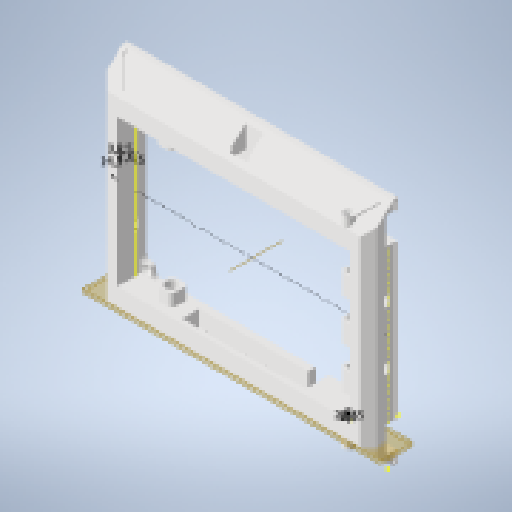
# Autodesk Inventor part: up_part
Saved by Autodesk Inventor 2025 (Build 290162000, 162)
## iProperties
Created: 2026-07-31
Part Number: up_part
Material: Типовые
Document SubType Name: Modeling
Designer: garin
Density: 1 g/cm^3
Appearance: По умолчанию
Author: garin
Autodesk Inventor part; units mm, degrees
ref_plane "YZ Plane" through (0, 0, 0) normal (1, 0, 0) x (0, 1, 0)
ref_plane "XZ Plane" through (0, 0, 0) normal (0, 1, 0) x (-1, 0, 0)
ref_plane "XY Plane" through (0, 0, 0) normal (0, 0, 1) x (1, 0, 0)
sketch "Эскиз1" plane through (0, 0, 0) normal (0, 0, 1) x (1, 0, 0)
  line L0 (0, 0) -> (-157, 0)
  line L1 (-157, 0) -> (-157, 133.4)
  line L2 (-157, 133.4) -> (0, 133.4)
  line L3 (0, 133.4) -> (0, 0)
  line L4 (-157, 66.7) -> (0, 66.7) construction
  line L5 (-78.5, 0) -> (-78.5, 133.4) construction
  line L6 (-11, 24.1) -> (-146, 24.1)
  line L7 (-146, 24.1) -> (-146, 109.3)
  line L8 (-146, 109.3) -> (-11, 109.3)
  line L9 (-11, 109.3) -> (-11, 24.1)
  line L10 (-11, 24.1) -> (-146, 109.3) construction
  line L11 (-146, 24.1) -> (-11, 109.3) construction
  line L12 (0, 0) -> (-2, 0) construction
  line L13 (-2, 0) -> (-2, 54.105) construction
  line L14 (-2, 54.105) -> (0, 54.105) construction
  line L15 (0, 54.105) -> (0, 0) construction
  line L16 (-2, 54.105) -> (-2, 73.295)
  line L17 (-2, 73.295) -> (-11, 73.295)
  line L18 (-2, 54.105) -> (-11, 54.105)
  line L19 (-157, 133.4) -> (-137, 133.4) construction
  line L20 (-157, 110.4) -> (-157, 133.4) construction
  line L21 (-157, 0) -> (-140, 0)
  line L22 (-140, 0) -> (-140, 22)
  line L23 (-140, 22) -> (-157, 22)
  line L24 (-157, 22) -> (-157, 0)
  line L25 (-157, 0) -> (-140, 0)
  line L26 (-140, 0) -> (-140, 6.5)
  line L27 (-140, 6.5) -> (-157, 6.5)
  line L28 (-157, 6.5) -> (-157, 0)
  line L29 (-140, 133.4) -> (-140, 111.4)
  line L30 (-140, 111.4) -> (-157, 111.4)
  line L31 (-140, 126.9) -> (-157, 126.9)
  line L32 (-17, 0) -> (-17, 22)
  line L33 (-17, 22) -> (0, 22)
  line L34 (-17, 6.5) -> (0, 6.5)
  line L35 (-17, 111.4) -> (0, 111.4)
  line L36 (-17, 126.9) -> (0, 126.9)
  line L37 (-17, 133.4) -> (-17, 111.4)
  point P0 (-78.5, 66.7)
  point P1 (0, 111.4)
  point P2 (0, 126.9)
  point P3 (-17, 126.9)
  point P4 (-140, 126.9)
  point P5 (0, 6.5)
  dimension "d0" = 157
  dimension "d1" = 133.4
  dimension "d2" = 135
  dimension "d3" = 85.2
  dimension "d20" = 2
  dimension "d21" = 54.105
  dimension "d22" = 19.19
  dimension "d75" = 17
  dimension "d76" = 22
  dimension "d77" = 17
  dimension "d78" = 6.5
  constraints: 76 end point, 15 symmetric about line, 10 parallel, 7 midpoint, 7 perpendicular, 6 horizontal, 2 point on line, 1 vertical
  measures "d0" distance of L1.end L2.end
  measures "d1" distance of L0.end L1.end
  measures "d2" distance of L7.end L8.end
  measures "d3" distance of L6.end L7.end
  measures "d20" distance of L13.end L14.end
  measures "d21" distance of L12.end L13.end
  measures "d22" distance of L13.end L16.end
  measures "d75" distance of L23.end L22.end
  measures "d76" distance of L22.end L21.end
  measures "d77" distance of L27.end L26.end
  measures "d78" distance of L26.end L25.end
extrude "Выдавливание1" add sketch "Эскиз1" along normal blind 17 contours L0 L32 L34 L3 | L0 L22 L23 L1 L30 L29 L2 L37 L35 L3 L33 L32 | L34 L32 L33 L3 | L0 L1 L27 L22 | L27 L1 L23 L22 | L35 L37 L36 L3 | L36 L37 L2 L3 | L1 L31 L29 L30 | L1 L2 L29 L31 | L9 L17 L16 L18
chamfer "Фаска1" distance 14 angle 45 2 edges at (-78.5, 0, 17) (-78.5, 133.4, 17)
chamfer "Фаска2" distance 5 angle 45 2 edges at (-157, 66.7, 17) (0, 66.7, 17)
sketch "Эскиз2" plane through (-157, 0, 3) normal (0, -0.7071068, 0.7071068) x (1, 0, 0)
  line L0 (0, -2.1213) -> (157, -2.1213) projected
  line L1 (0, -2.1213) -> (157, -2.1213)
  line L2 (157, -2.1213) -> (157, 19.7987)
  line L3 (157, 19.7987) -> (0, 19.7987)
  line L4 (0, 19.7987) -> (0, -2.1213)
  line L5 (78.5, 19.7987) -> (78.5, -2.1213) construction
  line L6 (0, 8.8387) -> (157, 8.8387) construction
  line L7 (154, 1.3387) -> (3, 1.3387) construction
  line L8 (3, 1.3387) -> (3, 16.3387) construction
  line L9 (3, 16.3387) -> (154, 16.3387) construction
  line L10 (154, 16.3387) -> (154, 1.3387) construction
  line L11 (154, 1.3387) -> (3, 16.3387) construction
  line L12 (3, 1.3387) -> (154, 16.3387) construction
  line L13 (3, 16.3387) -> (12, 16.3387) construction
  line L14 (12, 16.3387) -> (3, 3.6108)
  line L15 (0, 12.7279) -> (5, 19.799) construction
  line L16 (145, 16.3387) -> (154, 3.6108)
  line L17 (12, 16.3387) -> (145, 16.3387)
  line L18 (11, 14.92) -> (11, 26.9408) projected
  line L19 (154, 3.6108) -> (154, 1.3387)
  line L20 (154, 1.3387) -> (3, 1.3387)
  line L21 (3, 3.6108) -> (3, 1.3387)
  line L22 (5.2571, 3.3387) -> (13.0353, 14.3387)
  line L23 (13.0353, 14.3387) -> (143.9647, 14.3387)
  line L24 (143.9647, 14.3387) -> (151.7429, 3.3387)
  line L25 (151.7429, 3.3387) -> (5.2571, 3.3387)
  point P0 (78.5, 8.8387)
  dimension "d12" = 157
  dimension "d13" = 21.92
  dimension "d14" = 151
  dimension "d15" = 15
  dimension "d16" = 9
  dimension "d17" = 2
  constraints: 46 end point, 7 midpoint, 5 parallel, 5 perpendicular, 2 horizontal, 2 point on line, 2 symmetric about line, 1 collinear, 3 other
  measures "d12" distance of L3.end L2.end
  measures "d13" distance of L2.end L1.end
  measures "d14" distance of L8.end L9.end
  measures "d15" distance of L7.end L8.end
  measures "d16" distance of L8.end L13.end
  measures "d17" distance between parallel lines of L14 L22
extrude "Выдавливание2" cut sketch "Эскиз2" against normal blind 1 contours L17 L16 L19 L20 L21 L14
ref_plane "РабПлоскость1" through (-157, 66.7, 0) normal (0, 1, 0) x (1, 0, 0)
mirror "Зеркальное отражение1" about plane through (-157, 66.7, 0) normal (0, 1, 0) of "Выдавливание2"
extrude "Выдавливание3" cut sketch "Эскиз1" along normal blind 11.1 contours L9 L17 L16 L18
sketch "Эскиз3" plane through (-157, 0, 0) normal (0, -1, 0) x (1, 0, 0)
  line L0 (0, 0) -> (157, 0) construction
  line L1 (0, 0) -> (157, 0) construction
  line L2 (157, 0) -> (157, 17) construction
  line L3 (157, 17) -> (0, 17) construction
  line L4 (0, 17) -> (0, 0) construction
  line L5 (78.5, 17) -> (78.5, 0) construction
  line L6 (0, 8.5) -> (157, 8.5) construction
  line L7 (145, 14.5532) -> (12, 14.5532) construction
  line L8 (12, 14.5532) -> (12, 3.9466) construction
  line L9 (3, 3.9466) -> (154, 3.9466) construction
  line L10 (12, 9.2499) -> (78.5, 9.2499) construction
  line L11 (12, 9.2499) -> (78.5, 9.2499) construction
  line L12 (83.5, 4.2499) -> (73.5, 4.2499)
  line L13 (73.5, 4.2499) -> (73.5, 14.2499)
  line L14 (73.5, 14.2499) -> (83.5, 14.2499)
  line L15 (83.5, 14.2499) -> (83.5, 4.2499)
  line L16 (83.5, 4.2499) -> (73.5, 14.2499) construction
  line L17 (73.5, 4.2499) -> (83.5, 14.2499) construction
  line L18 (46.5, 13.7499) -> (108.5, 13.7499) construction
  line L19 (108.5, 13.7499) -> (108.5, 4.7499) construction
  line L20 (108.5, 4.7499) -> (46.5, 4.7499) construction
  line L21 (46.5, 4.7499) -> (46.5, 13.7499) construction
  line L22 (46.5, 13.7499) -> (108.5, 4.7499) construction
  line L23 (108.5, 13.7499) -> (46.5, 4.7499) construction
  line L24 (109, 14.2499) -> (46, 14.2499)
  line L25 (46, 14.2499) -> (46, 4.2499)
  line L26 (46, 4.2499) -> (109, 4.2499)
  line L27 (109, 4.2499) -> (109, 14.2499)
  line L28 (46.5, 9.2499) -> (48.3, 9.2499) construction
  line L29 (48.3, 7.2499) -> (48.3, 11.2499) construction
  circle A0 centre (48.3, 11.2499) radius 1.75
  circle A1 centre (48.3, 7.2499) radius 1.75
  line L30 (109, 14.2499) -> (117, 14.2499)
  line L31 (117, 14.2499) -> (117, 4.2499)
  line L32 (117, 4.2499) -> (109, 4.2499)
  line L33 (109, 4.2499) -> (109, 14.2499)
  line L34 (108.5, 13.7499) -> (98.75, 13.7499) construction
  line L35 (98.75, 13.7499) -> (98.75, 11.6499) construction
  line L36 (98.75, 11.6499) -> (108.5, 11.6499) construction
  line L37 (108.5, 11.6499) -> (108.5, 13.7499) construction
  circle A2 centre (98.75, 11.6499) radius 1.75
  line L38 (78.5, 9.2499) -> (77.5, 9.2499) construction
  line L39 (97, 11.6499) -> (97, 14.2499) construction
  line L40 (97, 14.2499) -> (95.5, 14.2499) construction
  line L41 (95.5, 14.2499) -> (95.5, 4.2499)
  line L42 (95.5, 4.2499) -> (97, 4.2499) construction
  line L43 (97, 4.2499) -> (97, 14.2499) construction
  line L44 (83.5, 14.2499) -> (84.5, 14.2499) construction
  line L45 (84.5, 14.2499) -> (84.5, 4.2499)
  line L46 (84.5, 4.2499) -> (83.5, 4.2499) construction
  line L47 (83.5, 4.2499) -> (83.5, 14.2499) construction
  line L48 (73.5, 14.2499) -> (71.5, 14.2499) construction
  line L49 (71.5, 14.2499) -> (71.5, 4.2499)
  line L50 (71.5, 4.2499) -> (73.5, 4.2499) construction
  line L51 (73.5, 4.2499) -> (73.5, 14.2499) construction
  line L52 (46, 14.2499) -> (50.15, 14.2499) construction
  line L53 (50.15, 14.2499) -> (50.15, 4.2499)
  line L54 (50.15, 4.2499) -> (46, 4.2499) construction
  line L55 (46, 4.2499) -> (46, 14.2499) construction
  line L56 (117, 4.2499) -> (109, 4.2499)
  line L57 (109, 4.2499) -> (109, -0.0001)
  line L58 (109, -0.0001) -> (117, -0.0001)
  line L59 (117, -0.0001) -> (117, 4.2499)
  point P0 (50.15, 14.2499)
  point P1 (50.15, 4.2499)
  point P2 (71.5, 4.2499)
  point P3 (71.5, 14.2499)
  dimension "d41" = 3.5
  dimension "d25" = 157
  dimension "d26" = 17
  dimension "d28" = 10
  dimension "d29" = 10
  dimension "d30" = 62
  dimension "d31" = 9
  dimension "d32" = 0.5
  dimension "d33" = 1.8
  dimension "d34" = 4
  dimension "d35" = 3.5
  dimension "d36" = 3.5
  dimension "d37" = 8
  dimension "d38" = 10
  dimension "d39" = 9.75
  dimension "d40" = 2.1
  dimension "d42" = 1
  dimension "d44" = 1.5
  dimension "d45" = 10
  dimension "d46" = 1
  dimension "d47" = 10
  dimension "d48" = 2
  dimension "d49" = 10
  dimension "d50" = 4.15
  dimension "d51" = 10
  dimension "d63" = 8
  dimension "d64" = 4.25
  constraints: 114 end point, 23 parallel, 12 horizontal, 12 perpendicular, 11 midpoint, 8 point on line, 3 coincident, 3 vertical, 2 centre point, 1 collinear, 1 horizontal alignment, 5 other
  measures "d25" distance of L3.end L2.end
  measures "d26" distance of L2.end L1.end
  measures "d28" distance of L13.end L14.end
  measures "d29" distance of L12.end L13.end
  measures "d30" distance of L19.end L20.end
  measures "d31" distance of L18.end L19.end
  measures "d32" distance between parallel lines of L18 L24
  measures "d33" distance of L28.end L28.start
  measures "d34" distance of L29.start L29.end
  measures "d35" diameter of A0
  measures "d36" diameter of A1
  measures "d37" distance of L31.end L32.end
  measures "d38" distance of L30.end L31.end
  measures "d39" distance of L36.end L35.end
  measures "d40" distance of L35.end L34.end
  measures "d42" distance of L11.end L38.end
  measures "d44" distance of L42.end L41.end
  measures "d45" distance of L41.end L40.end
  measures "d46" distance of L45.end L46.end
  measures "d47" distance of L44.end L45.end
  measures "d48" distance of L50.end L49.end
  measures "d49" distance of L49.end L48.end
  measures "d50" distance of L53.end L54.end
  measures "d51" distance of L52.end L53.end
  measures "d63" distance of L58.end L57.end
  measures "d64" distance of L57.end L56.end
extrude "Выдавливание4" cut sketch "Эскиз3" along normal blind 25 from surface at -24.1 contours L12 L13 L14 L15
ref_plane "РабПлоскость4" through (-145, 12.2603, 13.8461) normal (0, 1, 0) x (1, 0, 0)
ref_plane "РабПлоскость5" through (-145, 15.0603, 13.8461) normal (0, 1, 0) x (1, 0, 0)
extrude "Выдавливание5" cut sketch "Эскиз3" against normal blind 13 from surface at -12.2603 contours L27 L30 L31 L32 | L32 L59 L58 L57
extrude "Выдавливание6" cut sketch "Эскиз3" against normal blind 10 from surface at -15.0603 contours L12 L13 L14 L15 | L15 L24 L45 L26 | L26 L49 L24 L13 | L45 L24 L41 L26 | L26 L53 L24 L49 | L41 L24 L27 L26 | L26 L25 L24 L53 | A0 | A1 | A2
extrude "Выдавливание7" cut sketch "Эскиз3" along normal blind 3 from surface at -15.0603 contours A0 | A1 | A2
extrude "Выдавливание8" cut sketch "Эскиз3" along normal blind 2 from surface at -15.0603 contours L45 L24 L41 L26 | L26 L53 L24 L49
pattern_circular "Круговой массив1" count 2 over 360 about axis through (-78.5, 66.7, 0) along (0, 0, -1) of "Выдавливание4", "Выдавливание8", "Выдавливание6", "Выдавливание7", "Выдавливание5"
chamfer "Фаска3" distance 2 angle 45 1 edges at (-2, 63.7, 11.1)
sketch "Эскиз5" plane through (0, 0, 0) normal (1, 0, 0) x (0, 0, -1)
  line L0 (-12, 9) -> (-12, 124.4) projected
  line L1 (-3, 0) -> (-12, 9) projected
  line L2 (0, 0) -> (-3, 0) projected
  line L3 (0, 0) -> (0, 133.4) projected
  line L4 (0, 133.4) -> (-3, 133.4) projected
  line L5 (-12, 124.4) -> (-3, 133.4) projected
  line L6 (-11, 123.9858) -> (-11, 9.4142)
  line L7 (-11, 9.4142) -> (-2.5858, 1)
  line L8 (-2.5858, 1) -> (-1, 1)
  line L9 (-1, 1) -> (-1, 132.4)
  line L10 (-1, 132.4) -> (-2.5858, 132.4)
  line L11 (-2.5858, 132.4) -> (-11, 123.9858)
  line L12 (-10, 9.8284) -> (-10, 123.5716)
  line L13 (-10, 123.5716) -> (-2, 131.5716)
  line L14 (-2, 131.5716) -> (-2, 1.8284)
  line L15 (-2, 1.8284) -> (-10, 9.8284)
  dimension "d81" = 1
  dimension "d82" = 1
  constraints: 20 end point, 8 other
  measures "d81" distance between parallel lines of L0 L6
  measures "d82" distance between parallel lines of L6 L12
extrude "Выдавливание11" cut sketch "Эскиз1" along normal blind 6 contours L34 L32 L33 L3 | L27 L1 L23 L22 | L35 L37 L36 L3 | L1 L31 L29 L30
extrude "Выдавливание12" cut sketch "Эскиз5" against normal blind 1 contours L11 L10 L9 L8 L7 L6 | L12 L13 L14 L15
chamfer "Фаска4" distance 1 angle 45 4 edges at (-9, 6.5, 6) (-9, 126.9, 6) (-148.5, 126.9, 6) (-148.5, 6.5, 6)
ref_plane "РабПлоскость6" through (-78.5, 22, 0) normal (1, 0, 0) x (0, 0, -1)
mirror "Зеркальное отражение3" about plane through (-78.5, 22, 0) normal (1, 0, 0) of "Выдавливание12"
ref_plane "РабПлоскость7" through (0, 0, 6) normal (0, 0, 1) x (1, 0, 0)
sketch "Эскиз6" plane through (0, 0, 6) normal (0, 0, 1) x (1, 0, 0)
  line L0 (0, 111.4) -> (0, 22) construction
  line L1 (0, 66.7) -> (-157, 66.7) construction
  line L2 (-157, 124.4) -> (-157, 9) construction
  line L3 (-157, 66.7) -> (-157, 81.2) construction
  line L4 (-146, 24.1) -> (-146, 109.3) construction
  line L5 (-157, 81.2) -> (-146, 81.2) construction
  line L6 (-146, 81.2) -> (-146, 86.2) construction
  line L7 (-146, 86.2) -> (-157, 86.2) construction
  line L8 (-157, 86.2) -> (-157, 81.2) construction
  line L9 (-157, 83.7) -> (-146, 83.7) construction
  line L10 (-157, 83.7) -> (-148.5, 83.7) construction
  circle A0 centre (-148.5, 83.7) radius 0.8
  circle A1 centre (-148.5, 49.7) radius 0.8
  line L11 (-157, 81.2) -> (-157, 81) construction
  line L12 (-157, 81) -> (-146, 81)
  line L13 (-157, 86.4) -> (-146, 86.4)
  line L14 (-146, 86.4) -> (-146, 81)
  line L15 (-146, 24.1) -> (-146, 109.3) projected
  line L16 (-157, 81) -> (-157, 86.4)
  line L17 (-157, 52.4) -> (-146, 52.4)
  line L18 (-157, 47) -> (-146, 47)
  line L19 (-146, 47) -> (-146, 52.4)
  line L20 (-157, 52.4) -> (-157, 47)
  point P0 (0, 0)
  dimension "d91" = 14.5
  dimension "d92" = 5
  dimension "d93" = 8.5
  dimension "d94" = 1.6
  dimension "d99" = 0.2
  constraints: 34 end point, 7 symmetric about line, 5 point on line, 4 midpoint, 2 centre point, 2 collinear, 2 parallel, 2 perpendicular, 1 coincident, 1 horizontal, 1 other
  measures "d91" distance of L1.end L3.end
  measures "d92" distance of L6.end L5.end
  measures "d93" distance of L9.start L10.end
  measures "d94" diameter of A0
  measures "d99" distance of L3.end L11.end
extrude "Выдавливание13" cut sketch "Эскиз6" along normal blind 4 and the other way blind 6 contours A0 | A1
extrude "Выдавливание14" cut sketch "Эскиз6" along normal mid plane 2.8 contours A0 | A1 | L16 L13 L14 L12 | L18 L20 L17 L15
chamfer "Фаска5" distance 0.9 angle 45 2 edges at (-149.3, 83.7, 0) (-149.3, 49.7, 0)
mirror "Зеркальное отражение4" about plane through (-78.5, 22, 0) normal (1, 0, 0) of "Выдавливание14", "Выдавливание13", "Фаска5"
ref_plane "РабПлоскость8" through (-146, 36.9, 17) normal (0, 1, 0) x (1, 0, 0)
sketch "Эскиз7" plane through (-146, 24.1, 17) normal (0, 1, 0) x (1, 0, 0)
  line L0 (135, 17) -> (135, 0) projected
  line L1 (135, 0) -> (131.45, 0) construction
  line L2 (131.45, 0) -> (131.45, 2.95) construction
  line L3 (131.45, 2.95) -> (135, 2.95) construction
  line L4 (135, 2.95) -> (135, 0) construction
  circle A0 centre (131.45, 2.95) radius 1.3
  circle A1 centre (131.45, 2.95) radius 2.95
  line L5 (131.45, 5.9) -> (135, 5.9)
  line L6 (135, 5.9) -> (135, 0)
  line L7 (131.45, 0) -> (135, 0)
  circle A2 centre (131.45, 2.95) radius 3.5
  point P0 (146, 17)
  dimension "d105" = 3.55
  dimension "d106" = 2.95
  dimension "d107" = 2.6
  dimension "d117" = 7
  constraints: 14 end point, 3 centre point, 3 coincident, 3 equal length, 3 perpendicular, 2 point on circle, 2 tangent, 1 horizontal, 1 point on line
  measures "d105" distance of L2.end L3.end
  measures "d106" distance of L1.end L2.end
  measures "d107" diameter of A0
  measures "d117" diameter of A2
extrude "Выдавливание15" add sketch "Эскиз7" along normal blind 11.6 from surface at 12.8 contours L0 L7 A2 L5 | A2 L7 A1 L5 | A1 picked at (134.7433, 3.1824)
pattern_linear "Прямоуг.массив1" count 3 spacing 24 along (0, 1, 0) of "Выдавливание15"
fillet "Сопряжение2" radius 2 2 edges at (-11, 42.7, 11.1) (-11, 90.7, 11.1)
ref_plane "РабПлоскость10" through (-5, 14, 17) normal (0, 1, 0) x (1, 0, 0)
extrude "Выдавливание16" cut sketch "Эскиз7" against normal blind 20 contours A0
extrude "Выдавливание17" add sketch "Эскиз7" against normal blind 5.9 from surface at -10.1 contours A1
chamfer "Фаска6" distance 1.65 angle 45 1 edges at (-15.85, 8.1, 14.05)
mirror "Зеркальное отражение5" about plane through (-157, 66.7, 0) normal (0, 1, 0) of "Выдавливание17", "Фаска6", "Выдавливание16"
sketch "Эскиз9" plane through (-146, 24.1, 17) normal (0, 1, 0) x (1, 0, 0)
  line L0 (106, 3.1539) -> (106, 2.7501) projected
  line L1 (106, 17) -> (106, 3.1539) projected
  line L2 (106, 2.7501) -> (106, 17)
  line L3 (39.15, 2.7501) -> (35, 2.7501) projected
  line L4 (35, 2.7501) -> (35, 17) construction
  line L5 (-11, 17) -> (146, 17) projected
  line L6 (35, 9.8751) -> (22, 9.8751) construction
  line L7 (27, 4.8751) -> (17, 4.8751)
  line L8 (17, 4.8751) -> (17, 14.8751)
  line L9 (17, 14.8751) -> (27, 14.8751)
  line L10 (27, 14.8751) -> (27, 4.8751)
  line L11 (27, 4.8751) -> (17, 14.8751) construction
  line L12 (17, 4.8751) -> (27, 14.8751) construction
  circle A0 centre (22, 9.8751) radius 3.6
  dimension "d135" = 13
  dimension "d136" = 10
  dimension "d137" = 10
  dimension "d138" = 7.2
  constraints: 18 end point, 3 midpoint, 2 horizontal, 2 parallel, 1 centre point, 1 coincident, 1 collinear, 1 perpendicular, 1 point on line, 1 vertical
  measures "d135" distance of L6.start L6.end
  measures "d136" distance of L8.end L9.end
  measures "d137" distance of L7.end L8.end
  measures "d138" diameter of A0
extrude "Выдавливание19" add sketch "Эскиз9" along normal blind 7
fillet "Сопряжение3" radius 3 4 edges at (-129, 27.6, 12.1249) (-129, 27.6, 2.1249) (-119, 27.6, 12.1249) (-119, 27.6, 2.1249)
mirror "Зеркальное отражение6" about plane through (-157, 66.7, 0) normal (0, 1, 0) of "Сопряжение3", "Выдавливание19"
sketch "Эскиз10" plane through (0, 0, 0) normal (0, 0, -1) x (-1, 0, 0)
  line L0 (146, 109.3) -> (11, 109.3) projected
  line L1 (146, 109.3) -> (140, 109.3)
  line L2 (140, 109.3) -> (140, 103.3)
  line L3 (140, 103.3) -> (146, 103.3)
  line L4 (146, 103.3) -> (146, 109.3)
  line L5 (143, 109.3) -> (143, 103.3) construction
  line L6 (140, 106.3) -> (146, 106.3) construction
  circle A0 centre (143, 106.3) radius 1.25
  line L7 (78.5, 109.3) -> (78.5, 24.1) construction
  line L8 (48, 24.1) -> (146, 24.1) construction
  line L9 (13.25, 72.5) -> (13.25, 60.9) construction
  line L10 (13.25, 66.7) -> (146, 66.7) construction
  line L11 (146, 24.1) -> (146, 109.3) construction
  line L12 (11, 109.3) -> (17, 109.3)
  line L13 (17, 109.3) -> (17, 103.3)
  line L14 (17, 103.3) -> (11, 103.3)
  line L15 (11, 103.3) -> (11, 109.3)
  line L16 (14, 109.3) -> (14, 103.3) construction
  line L17 (17, 106.3) -> (11, 106.3) construction
  circle A1 centre (14, 106.3) radius 1.25
  line L18 (11, 24.1) -> (11, 109.3) construction
  line L19 (146, 24.1) -> (140, 24.1)
  line L20 (140, 24.1) -> (140, 30.1)
  line L21 (140, 30.1) -> (146, 30.1)
  line L22 (146, 30.1) -> (146, 24.1)
  line L23 (143, 24.1) -> (143, 30.1) construction
  line L24 (140, 27.1) -> (146, 27.1) construction
  circle A2 centre (143, 27.1) radius 1.25
  line L25 (146, 109.3) -> (146, 24.1) construction
  line L26 (17, 27.1) -> (11, 27.1) construction
  circle A3 centre (14, 27.1) radius 1.25
  line L27 (17, 24.1) -> (17, 30.1)
  line L28 (17, 30.1) -> (11, 30.1)
  line L29 (11, 30.1) -> (11, 24.1)
  line L30 (14, 24.1) -> (14, 30.1) construction
  line L31 (11, 24.1) -> (17, 24.1)
  point P0 (0, 0)
  dimension "d142" = 6
  dimension "d143" = 6
  dimension "d144" = 2.5
  constraints: 56 end point, 27 symmetric about line, 8 midpoint, 4 centre point, 2 parallel, 1 horizontal, 1 perpendicular, 1 point on line, 1 vertical, 3 other
  measures "d142" distance of L3.end L2.end
  measures "d143" distance of L2.end L1.end
  measures "d144" diameter of A0
extrude "Выдавливание20" add sketch "Эскиз10" against normal blind 3
chamfer "Фаска7" distance 1.5 angle 45 4 edges at (-141.75, 106.3, 3) (-141.75, 27.1, 3) (-12.75, 27.1, 3) (-12.75, 106.3, 3)
fillet "Сопряжение4" radius 2.5 12 edges at (-17, 109.3, 1.5) (-17, 103.3, 1.5) (-11, 103.3, 1.5) (-11, 30.1, 1.5) (-17, 30.1, 1.5) (-17, 24.1, 1.5) (-140, 24.1, 1.5) (-140, 30.1, 1.5) (-146, 30.1, 1.5) (-146, 103.3, 1.5) (-140, 103.3, 1.5) (-140, 109.3, 1.5)
